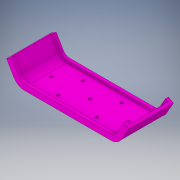
# Autodesk Inventor part: Drill Helper v 1
Saved by Autodesk Inventor 2019 (Build 230136000, 136)
## iProperties
Created: 2021-07-21
Part Number: Drill Helper v 1
Material: Generic
Document SubType Name: Modeling
Designer: Lix
Density: 1 g/cm^3
Appearance: Magenta
Author: Lix
Autodesk Inventor part; units mm, degrees
ref_plane "YZ Plane" through (0, 0, 0) normal (1, 0, 0) x (0, 1, 0)
ref_plane "XZ Plane" through (0, 0, 0) normal (0, 1, 0) x (-1, 0, 0)
ref_plane "XY Plane" through (0, 0, 0) normal (0, 0, 1) x (1, 0, 0)
sketch "Sketch1" plane through (0, 0, 0) normal (0, 0, 1) x (1, 0, 0)
  arc A0 (-53.4049, 8) -> (-44.7446, 3) centre (-44.7446, 13) ccw
  line L0 (-44.7446, 3) -> (44.7446, 3)
  arc A1 (44.7446, 3) -> (53.4049, 8) centre (44.7446, 13) ccw
  line L1 (53.4049, 8) -> (60.8108, 20.8273)
  line L2 (-60.8108, 20.8273) -> (-53.4049, 8)
  line L3 (63.4088, 19.3273) -> (56.003, 6.5)
  arc A2 (44.7446, 0) -> (56.003, 6.5) centre (44.7446, 13) ccw
  line L4 (44.7446, 0) -> (-44.7446, 0)
  arc A3 (-56.003, 6.5) -> (-44.7446, 0) centre (-44.7446, 13) ccw
  line L5 (-56.003, 6.5) -> (-63.4088, 19.3273)
  line L6 (-63.4088, 19.3273) -> (-60.8108, 20.8273)
  line L7 (-60.8108, 20.8273) -> (60.8108, 20.8273) construction
  line L8 (-63.4088, 19.3273) -> (63.4088, 19.3273) construction
  line L9 (60.8108, 20.8273) -> (63.4088, 19.3273)
  point P0 (0, 0)
  point P1 (0, 0)
  constraints: 20 end point, 8 point on circle, 4 centre point, 2 parallel, 1 horizontal, 1 midpoint, 1 perpendicular, 2 other
extrude "Extrusion1" add sketch "Sketch1" along normal blind 40
sketch "Sketch2" plane through (-44.7446, 0, 0) normal (0, -1, 0) x (1, 0, 0)
  line L0 (89.4893, 0) -> (0, 0) projected
  line L1 (-11.2583, 0) -> (-11.2583, 40) projected
  point P0 (44.7446, 0)
  point P1 (4.7446, 20)
  point P2 (44.7446, 20)
  point P3 (84.7446, 20)
  point P4 (44.7446, 0)
  point P5 (-11.2583, 20)
  dimension "d3" = 40
  dimension "d4" = 40
  constraints: 3 horizontal alignment, 2 midpoint, 1 vertical alignment
  measures "d3" distance of point (44.745, 20) point (4.745, 20)
  measures "d4" distance of point (84.745, 20) point (44.745, 20)
hole "Hole1" at (-40, 0, 20) at (0, 0, 20) at (40, 0, 20) direction (0, 1, 0) diameter 3 end through all
sketch "Sketch3" plane through (-44.7446, 0, 0) normal (0, -1, 0) x (1, 0, 0)
  circle A0 centre (44.7446, 20) radius 1.5 projected
  line L0 (89.4893, 0) -> (0, 0) projected
  line L1 (0, 0) -> (0, 40) projected
  line L2 (0, 20) -> (89.4893, 20) construction
  line L3 (89.4893, 0) -> (89.4893, 40) projected
  point P0 (44.7446, 0)
  point P1 (24.7446, 7)
  point P2 (64.7446, 7)
  point P3 (24.7446, 33)
  point P4 (64.7446, 33)
  dimension "d12" = 20
  dimension "d13" = 20
  dimension "d14" = 7
  constraints: 2 end point, 2 midpoint, 2 symmetric about line, 1 horizontal alignment
  measures "d12" horizontal distance of point (24.745, 7) A0.centre
  measures "d13" horizontal distance of A0.centre point (64.745, 7)
  measures "d14" distance from line of L0 point (24.745, 7)
hole "Hole2" at (-20, 0, 7) at (20, 0, 7) at (-20, 0, 33) at (20, 0, 33) direction (0, 1, 0) diameter 3 end through all
ref_plane "Work Plane2" through (0, 0, 20) normal (0, 0, 1) x (1, 0, 0)
sketch "Sketch5" plane through (0, 0, 40) normal (0, 0, 1) x (1, 0, 0)
  arc A0 (-53.4049, 8) -> (-44.7446, 3) centre (-44.7446, 13) ccw projected
  line L0 (-53.4049, 8) -> (-60.8108, 20.8273) projected
  line L1 (-60.8108, 20.8273) -> (-63.4088, 19.3273) projected
  line L2 (-63.4088, 19.3273) -> (-56.003, 6.5) projected
  arc A1 (-56.003, 6.5) -> (-44.7446, 0) centre (-44.7446, 13) ccw projected
  line L3 (-44.7446, 0) -> (44.7446, 0) projected
  arc A2 (44.7446, 0) -> (56.003, 6.5) centre (44.7446, 13) ccw projected
  line L4 (56.003, 6.5) -> (63.4088, 19.3273) projected
  line L5 (63.4088, 19.3273) -> (60.8108, 20.8273) projected
  line L6 (60.8108, 20.8273) -> (53.4049, 8) projected
  arc A3 (44.7446, 3) -> (53.4049, 8) centre (44.7446, 13) ccw projected
  line L7 (44.7446, 3) -> (-44.7446, 3) projected
  point P0 (0, 0)
extrude "Extrusion3" add sketch "Sketch5" along normal blind 0.25
sketch "Sketch6" plane through (0, 0, 40.25) normal (0, 0, 1) x (1, 0, 0)
  arc A0 (-53.4049, 8) -> (-44.7446, 3) centre (-44.7446, 13) ccw projected
  line L0 (-53.4049, 8) -> (-60.8108, 20.8273) projected
  line L1 (-60.8108, 20.8273) -> (-63.4088, 19.3273) projected
  line L2 (-63.4088, 19.3273) -> (-56.003, 6.5) projected
  arc A1 (-56.003, 6.5) -> (-44.7446, 0) centre (-44.7446, 13) ccw projected
  line L3 (-44.7446, 0) -> (44.7446, 0) projected
  arc A2 (44.7446, 0) -> (56.003, 6.5) centre (44.7446, 13) ccw projected
  line L4 (56.003, 6.5) -> (63.4088, 19.3273) projected
  line L5 (63.4088, 19.3273) -> (60.8108, 20.8273) projected
  line L6 (60.8108, 20.8273) -> (53.4049, 8) projected
  arc A3 (44.7446, 3) -> (53.4049, 8) centre (44.7446, 13) ccw projected
  line L7 (44.7446, 3) -> (-44.7446, 3) projected
  arc A4 (-50.8068, 9.5) -> (-44.7446, 6) centre (-44.7446, 13) ccw
  line L8 (-50.8068, 9.5) -> (-58.2127, 22.3273)
  line L9 (58.2127, 22.3273) -> (50.8068, 9.5)
  arc A5 (44.7446, 6) -> (50.8068, 9.5) centre (44.7446, 13) ccw
  line L10 (44.7446, 6) -> (-44.7446, 6)
  line L11 (-63.4088, 19.3273) -> (-60.8108, 20.8273) projected
  line L12 (-63.4088, 19.3273) -> (-58.2127, 22.3273)
  line L13 (63.4088, 19.3273) -> (58.2127, 22.3273)
  dimension "d27" = 3
  constraints: 10 end point, 4 point on circle, 2 centre point, 1 perpendicular, 1 point on line, 1 other
  measures "d27" distance between parallel lines of L7 L10
extrude "Extrusion4" add sketch "Sketch6" along normal blind 3
mirror "Mirror2" about plane through (0, 0, 20) normal (0, 0, 1) of "Extrusion3", "Extrusion4"
equation "\"d4\" = d3"
equation "\"d13\" = d12"
body "Solid1"
